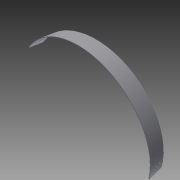
# Autodesk Inventor part: curvedTrack
Saved by Autodesk Inventor 2011 SP1 (Build 150282100, 282)
## iProperties
Created: 2013-01-18
Part Number: curvedTrack
Document SubType Name: Modeling
Designer: wes
Density: 1 g/cm^3
Author: wes
Autodesk Inventor part; units mm, degrees
ref_plane "YZ Plane" through (0, 0, 0) normal (1, 0, 0) x (0, 1, 0)
sketch "Sketch1" plane through (0, 0, 0) normal (0, 0, 1) x (1, 0, 0)
  arc A0 (380.5355, -38.0375) -> (-270.1768, 230.7579) centre (4.8231, -25.5444) ccw
  arc A1 (383.5416, -39.2939) -> (-271.6172, 233.6803) centre (4.8231, -25.5444) ccw
  line L0 (-271.6172, 233.6803) -> (-270.1768, 230.7579)
  line L1 (380.5355, -38.0375) -> (383.5416, -39.2939)
  point P0 (0, 0)
  dimension "d0" = 375.92
  dimension "d1" = 138.92
  dimension "d3" = 138.92
  dimension "d4" = 378.968
  constraints: 4 end point, 4 point on circle, 2 centre point, 1 coincident
  measures "d0" radius of A0
  measures "d4" radius of A1
extrude "Extrusion1" add sketch "Sketch1" along normal blind 76.2
ref_plane "Work Plane3" through (383.5416, -39.2939, 0) normal (0.9993, -0.0363, 0) x (0.0363, 0.9993, 0)
ref_plane "Work Plane4" through (-271.6172, 233.6803, 0) normal (-0.7295, 0.684, 0) x (-0.684, -0.7295, 0)
sketch "Sketch2" plane through (383.5416, -39.2939, 0) normal (0.9993, -0.0363, 0) x (0.0363, 0.9993, 0)
  line L0 (249.0245, 76.2) -> (0, 76.2) projected
  line L1 (0, 0) -> (0, 76.2) projected
  line L2 (249.0245, 0) -> (0, 0) projected
  line L3 (249.0245, 0) -> (249.0245, 76.2) projected
  point P0 (25.3526, 0)
  point P1 (38.1, 57.15)
  point P2 (38.1, 38.1)
  point P3 (38.1, 19.05)
  dimension "d7" = 38.1
  dimension "d8" = 38.1
  dimension "d9" = 38.1
  dimension "d10" = 19.05
  dimension "d11" = 38.1
  dimension "d12" = 57.15
  measures "d7" distance from line of point (38.1, 57.15) L1
  measures "d8" distance from line of L1 point (38.1, 38.1)
  measures "d9" distance from line of L1 point (38.1, 19.05)
  measures "d10" distance from line of point (38.1, 57.15) L0
  measures "d11" distance from line of L0 point (38.1, 38.1)
  measures "d12" distance from line of point (38.1, 19.05) L0
sketch "Sketch3" plane through (-271.6172, 233.6803, 0) normal (-0.7295, 0.684, 0) x (-0.684, -0.7295, 0)
  line L0 (0, 0) -> (0, 76.2) projected
  line L1 (-378.968, 0) -> (0, 0) projected
  point P0 (-15.3344, 0)
  point P1 (-38.1, 19.05)
  point P2 (-38.1, 38.1)
  point P3 (-38.1, 57.15)
  point P4 (-249.0245, 0)
  dimension "d13" = 38.1
  dimension "d14" = 38.1
  dimension "d15" = 38.1
  dimension "d16" = 19.05
  dimension "d17" = 38.1
  dimension "d18" = 57.15
  measures "d13" distance from line of L0 point (-38.1, 19.05)
  measures "d14" distance from line of L0 point (-38.1, 38.1)
  measures "d15" distance from line of L0 point (-38.1, 57.15)
  measures "d16" distance from line of point (-38.1, 19.05) L1
  measures "d17" distance from line of point (-38.1, 38.1) L1
  measures "d18" distance from line of L1 point (-38.1, 57.15)
hole "Hole1" at (-245.5557, 261.4726, 57.15) at (-245.5557, 261.4726, 38.1) at (-245.5557, 261.4726, 19.05) direction (0.7295, -0.684, 0) diameter 6.35 depth 25.4 tip angle 118
hole "Hole2" at (384.924, -1.219, 57.15) at (384.924, -1.219, 38.1) at (384.924, -1.219, 19.05) direction (-0.9993, 0.0363, 0) diameter 6.35 depth 25.4 tip angle 118
thread "Thread1" size "1/4-20 UNC" class "2B" standard "ANSI Unified Screw Threads" full length
thread "Thread2" size "1/4-20 UNC" class "2B" standard "ANSI Unified Screw Threads" full length
thread "Thread3" size "1/4-20 UNC" class "2B" standard "ANSI Unified Screw Threads" full length
thread "Thread4" size "1/4-20 UNC" class "2B" standard "ANSI Unified Screw Threads" full length
thread "Thread5" size "1/4-20 UNC" class "2B" standard "ANSI Unified Screw Threads" full length
thread "Thread6" size "1/4-20 UNC" class "2B" standard "ANSI Unified Screw Threads" full length
equation "\"d3\" = d1"
body "Solid1"
